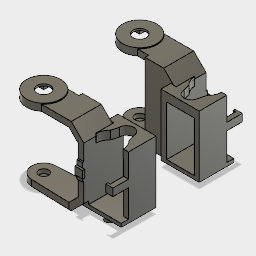
servo_bracket_knee_mirror (Autodesk Fusion 360 design; units mm, degrees)
Autodesk Fusion 360 part; units mm, degrees
sketch "スケッチ1" plane through (0, 0, 0) normal (0, 1, 0) x (1, 0, 0)
  circle A0 centre (0, 0) radius 5.55
  circle A1 centre (0, 0) radius 2.75
  line L0 (2.75, 2.75) -> (-2.75, 2.75)
  line L1 (-2.75, 2.75) -> (-2.75, -2.75)
  line L2 (-2.75, -2.75) -> (2.75, -2.75)
  line L3 (2.75, -2.75) -> (2.75, 2.75)
  line L4 (2.75, 2.75) -> (-2.75, -2.75) construction
  line L5 (-2.75, 2.75) -> (2.75, -2.75) construction
  line L6 (-2.75, 2.75) -> (-4.8208, 2.75)
  line L7 (-2.75, -2.75) -> (-4.8208, -2.75)
  line L8 (-2.75, 2.75) -> (-2.75, 4.8208)
  line L9 (-2.75, -2.75) -> (-2.75, -4.8208)
  line L10 (2.75, -2.75) -> (4.8208, -2.75)
  line L11 (2.75, -2.75) -> (2.75, -4.8208)
  line L12 (2.75, 2.75) -> (4.8208, 2.75)
  line L13 (2.75, 2.75) -> (2.75, 4.8208)
  dimension "d1" = 11.1
  dimension "d2" = 5.5
  dimension "d3" = 5.5
  dimension "d4" = 5.5
  constraint concentric A0 A1
  constraint perpendicular L0 L1
  constraint parallel L0 L2
  constraint parallel L1 L3
  constraint horizontal L0
  constraint coincident L4
  constraint coincident L5
  constraint coincident A0
  constraint perpendicular L1 L6
  constraint perpendicular L1 L7
  constraint perpendicular L7 L8
  constraint perpendicular L7 L9
  constraint perpendicular L9 L10
  constraint perpendicular L10 L11
  constraint perpendicular L11 L12
  constraint perpendicular L12 L13
  measures "d1" diameter of A0
  measures "d2" diameter of A1
sketch "スケッチ2" plane through (0, 0, 0) normal (0, 1, 0) x (1, 0, 0)
  circle A0 centre (0, 0) radius 7.15
  line L0 (5.5, 5.5) -> (-5.5, 5.5)
  line L1 (-5.5, 5.5) -> (-5.5, -5.5)
  line L2 (-5.5, -5.5) -> (5.5, -5.5)
  line L3 (5.5, -5.5) -> (5.5, 5.5)
  line L4 (5.5, 5.5) -> (-5.5, -5.5) construction
  line L5 (-5.5, 5.5) -> (5.5, -5.5) construction
  line L6 (0, 0) -> (22.2, 0)
  line L7 (5.5, -5.5) -> (5.5, 5.5)
  line L8 (5.5, 5.5) -> (22.2, 5.5)
  line L9 (22.2, 5.5) -> (22.2, -5.5)
  line L10 (22.2, -5.5) -> (5.5, -5.5)
  line L11 (22.2, -5.5) -> (19.88, -5.5)
  line L12 (19.88, -5.5) -> (19.88, 5.5)
  line L13 (19.88, 5.5) -> (22.2, 5.5)
  line L14 (22.2, 5.5) -> (22.2, -5.5)
  dimension "d5" = 14.3
  dimension "d6" = 11
  dimension "d7" = 11
  dimension "d8" = 22.2
  dimension "d9" = 2.32
  constraint perpendicular L0 L1
  constraint parallel L0 L2
  constraint parallel L1 L3
  constraint horizontal L0
  constraint coincident L4
  constraint coincident L5
  constraint perpendicular L7 L8
  constraint parallel L7 L9
  constraint parallel L8 L10
  constraint horizontal L11
  constraint vertical L12
  constraint horizontal L13
  measures "d5" diameter of A0
extrude "押し出し1" add sketch "スケッチ2" against normal blind 3 contours A0 L3 L6 L7 | A0 L3 L6 L7 | A0 L0 L1 L2 L3 L7 | A0 L0 | A0 L2 | A0 L1 makes body 1
extrude "押し出し2" cut sketch "スケッチ1" against normal blind 5.5 contours A0 L3 L10 L12 | A0 L0 L8 L13 | A1 L0 L3 | A0 L2 L9 L11 | A1 L2 L3 | A1 | A1 L0 L1 | A1 L1 L2 | A0 L1 L6 L7 bodies 1
extrude "押し出し3" add sketch "スケッチ1" against normal blind 0.8 contours A0 L3 L10 L12 | A0 L0 L8 L13 | A1 L0 L3 | A0 L2 L9 L11 | A1 L2 L3 | A1 L0 L1 | A1 L1 L2 | A0 L1 L6 L7 bodies 1
extrude "押し出し4" add sketch "スケッチ2" against normal blind 3 contours A0 L3 L6 L7 L10 L12 | A0 L3 L6 L7 L8 L12 | A0 L0 L3 L7 | A0 L2 L3 L7 bodies 1
extrude "押し出し5" add sketch "スケッチ2" against normal blind 32.7 contours L6 L8 L9 L12 L13 L14 | L6 L9 L10 L11 L12 L14 bodies 1
extrude "押し出し6" cut sketch "スケッチ2" against normal blind 0.4 contours A0 L3 L6 L7 L10 L12 | A0 L3 L6 L7 L8 L12 | A0 L0 L3 L7 | A0 L2 L3 L7 | L6 L8 L9 L12 L13 L14 | L6 L9 L10 L11 L12 L14 bodies 1
ref_plane "作業平面1" through (0, -32.7, 0) normal (0, 1, 0) x (1, 0, 0)
sketch "スケッチ3" plane through (0, -32.7, 0) normal (0, 1, 0) x (1, 0, 0)
  circle A0 centre (0, 0) radius 2
  circle A1 centre (0, 0) radius 5
  line L0 (0, 0) -> (16, 0)
  line L1 (16, 0) -> (16, 5.5)
  line L2 (16, 5.5) -> (-0.1554, 4.9976)
  line L3 (16, 5.5) -> (19.88, 5.5)
  line L4 (19.88, 5.5) -> (19.88, -5.5)
  line L5 (19.88, -5.5) -> (16, -5.5)
  line L6 (16, -5.5) -> (16, 0)
  line L7 (19.88, -5.5) -> (9.2, -5.5)
  line L8 (19.88, -5.5) -> (30.56, -5.5) construction
  line L9 (9.2, -5.5) -> (-0.2675, -4.9928)
  dimension "d23" = 4
  dimension "d24" = 10
  dimension "d25" = 16
  dimension "d26" = 180
  dimension "d27" = 10.68
  constraint perpendicular L0 L1
  constraint coincident A1
  constraint tangent A1 L2
  constraint perpendicular L1 L3
  constraint perpendicular L4 L5
  constraint horizontal L8
  constraint tangent A1 L9
  measures "d23" diameter of A0
  measures "d24" diameter of A1
  measures "d26" angle of L7 L8
extrude "押し出し7" add sketch "スケッチ3" along normal blind 2.6 bodies 1
extrude "押し出し8" add sketch "スケッチ3" along normal blind 0.8 contours A0 bodies 1
sketch "スケッチ4" plane through (0, 0, 0) normal (0, 1, 0) x (1, 0, 0)
  line L0 (22.2, -5.5) -> (22.2, -7)
  line L1 (22.2, -5.5) -> (23.7, -5.5) construction
  line L2 (22.2, -7) -> (9.2, -7)
  line L3 (22.2, -7) -> (35.2, -7) construction
  line L4 (9.2, -7) -> (9.2, -5.5)
  line L5 (9.2, -7) -> (9.2, -5.5)
  line L6 (22.2, -5.5) -> (9.2, -5.5)
  dimension "d32" = 90
  dimension "d33" = 1.5
  dimension "d34" = 180
  dimension "d35" = 13
  constraint horizontal L1
  constraint horizontal L3
  measures "d32" angle of L0 L1
  measures "d34" angle of L2 L3
extrude "押し出し9" add sketch "スケッチ4" against normal blind 32.7 bodies 1
extrude "押し出し10" cut sketch "スケッチ4" against normal blind 0.4 bodies 1
chamfer "面取り1" distance 3.88 angle 45 2 edges at (19.88, -3, 0) (19.88, -30.1, 0) on bodies 1
chamfer "面取り2" distance 5.2 angle 45 2 edges at (22.2, -0.4, 0.75) (22.2, -32.7, 0.75) on bodies 1
ref_plane "作業平面2" through (22.2, -16.55, 0.75) normal (1, 0, 0) x (0, 0, 1)
sketch "スケッチ5" plane through (22.2, -16.55, 0.75) normal (1, 0, 0) x (0, 0, -1)
  line L0 (6.25, -13.55) -> (-4.75, -13.55)
  line L1 (5.7476, -13.55) -> (-4.2428, -13.55)
  line L2 (-6.25, -10.95) -> (-6.25, -16.15)
  line L3 (-2.7394, -13.55) -> (-11.2658, -13.55)
  constraint coincident L0
  constraint perpendicular L2 L3
sketch "スケッチ6" plane through (22.2, -16.55, 0.75) normal (1, 0, 0) x (0, 0, -1)
  line L0 (-6.25, -10.95) -> (-6.25, -16.15)
  line L1 (-6.25, -13.55) -> (-6.25, -13.75)
  line L2 (-6.25, -13.55) -> (-6.05, -13.55) construction
  line L3 (-6.25, -13.75) -> (-10.25, -13.75)
  line L4 (-6.25, -13.75) -> (-2.25, -13.75) construction
  line L5 (-10.25, -13.75) -> (-6.25, -13.75)
  line L6 (-6.25, -13.75) -> (-6.25, 12.05)
  line L7 (-6.25, 12.05) -> (-10.25, 12.05)
  line L8 (-10.25, 12.05) -> (-10.25, -13.75)
  line L9 (-6.25, -13.75) -> (4.25, -13.75)
  line L10 (4.25, -13.75) -> (4.25, -12.25)
  line L11 (4.25, -12.25) -> (-6.25, -12.25)
  line L12 (-6.25, -12.25) -> (-6.25, -13.75)
  line L13 (-6.25, 12.05) -> (1.25, 12.05)
  line L14 (1.25, 12.05) -> (1.25, 8.55)
  line L15 (1.25, 8.55) -> (-6.25, 8.55)
  line L16 (-6.25, 8.55) -> (-6.25, 12.05)
  line L17 (-6.25, 8.55) -> (-10.25, 8.55)
  line L18 (-6.25, -12.25) -> (-10.25, -12.25)
  dimension "d43" = 90
  dimension "d44" = 0.2
  dimension "d45" = 180
  dimension "d46" = 4
  dimension "d47" = 25.8
  dimension "d48" = 10.5
  dimension "d49" = 1.5
  dimension "d50" = 7.5
  dimension "d51" = 3.5
  constraint midpoint L0
  constraint horizontal L2
  constraint horizontal L4
  constraint vertical L6
  constraint horizontal L7
  constraint vertical L8
  constraint horizontal L9
  constraint vertical L10
  constraint horizontal L11
  constraint vertical L12
  constraint horizontal L13
  constraint vertical L14
  constraint horizontal L15
  constraint vertical L16
  constraint coincident L8
  constraint perpendicular L8 L17
  constraint perpendicular L8 L18
  measures "d43" angle of L1 L2
  measures "d45" angle of L3 L4
extrude "押し出し11" add sketch "スケッチ6" along normal blind 2.32 separate body contours L0 L6 L8 L17 L18 makes body 2
extrude "押し出し12" add sketch "スケッチ6" along normal blind 15.92 contours L0 L1 L6 L9 L10 L11 L12 | L0 L1 L3 L5 L6 L8 L12 L18 | L6 L7 L8 L16 L17 | L6 L13 L14 L15 L16 bodies 2
extrude "押し出し13" cut sketch "スケッチ6" along normal blind 2.32 contours L0 L1 L6 L9 L10 L11 L12 | L6 L13 L14 L15 L16 bodies 2
sketch "スケッチ7" plane through (38.12, 0, 0) normal (1, 0, 0) x (0, 0, -1)
  line L0 (0.5, -4.5) -> (-11, -4.5)
  line L1 (-11, -4.5) -> (-11, -8)
  line L2 (-11, -8) -> (0.5, -8)
  line L3 (0.5, -8) -> (0.5, -4.5)
  line L4 (-11, -4.5) -> (0.5, -4.5)
  line L5 (0.5, -4.5) -> (0.5, -30.3)
  line L6 (0.5, -30.3) -> (-11, -30.3)
  line L7 (-11, -30.3) -> (-11, -4.5)
  dimension "d58" = 11.5
  dimension "d59" = 25.8
  constraint horizontal L4
  constraint vertical L5
  constraint horizontal L6
  constraint vertical L7
extrude "押し出し14" add sketch "スケッチ7" against normal blind 2 contours L2 L5 L6 L7 bodies 2
sketch "スケッチ8" plane through (0, -4.5, 0) normal (0, 1, 0) x (-1, 0, 0)
  line L0 (-24.52, 7) -> (-22.2, 7)
  line L1 (-22.2, 7) -> (-22.2, 11)
  line L2 (-22.2, 11) -> (-38.12, 11)
  line L3 (-38.12, 11) -> (-38.12, -0.5)
  line L4 (-38.12, -0.5) -> (-24.52, -0.5)
  line L5 (-24.52, -0.5) -> (-24.52, 7)
  line L6 (-24.52, -0.5) -> (-30.32, -0.5)
  line L7 (-24.52, -0.5) -> (-18.72, -0.5) construction
  circle A0 centre (-30.32, -0.5) radius 5.6
  line L8 (-30.32, -0.5) -> (-30.32, 6.5)
  line L9 (-30.32, -0.5) -> (-37.32, -0.5) construction
  circle A1 centre (-30.32, 6.5) radius 3
  line L10 (-30.32, 6.5) -> (-27.32, 6.5)
  line L11 (-30.32, 6.5) -> (-33.32, 6.5)
  line L12 (-27.32, 6.5) -> (-26.5193, 3.6127)
  line L13 (-27.32, 6.5) -> (-24.3238, 6.5) construction
  line L14 (-33.32, 6.5) -> (-34.1207, 3.6127)
  dimension "d62" = 180
  dimension "d63" = 5.8
  dimension "d64" = 11.2
  dimension "d65" = 90
  dimension "d66" = 7
  dimension "d67" = 6
  dimension "d68" = 74.5
  dimension "d69" = 105.5
  constraint horizontal L7
  constraint horizontal L9
  constraint coincident A1
  constraint perpendicular L8 L10
  constraint parallel L10 L11
  constraint coincident A0
  constraint horizontal L13
  measures "d62" angle of L6 L7
  measures "d64" diameter of A0
  measures "d65" angle of L8 L9
  measures "d67" diameter of A1
  measures "d68" angle of L12 L13
  measures "d69" angle of L13 L14
extrude "押し出し15" cut sketch "スケッチ8" against normal blind 7.5 contours L4 L6 A0 L8 A1 | L4 A0 L8 A1 | A0 A1 L12 | A0 L8 A1 | A0 L8 A1 | A0 L8 A1 L10 | A1 L10 L11 | A0 A1 L14 | A0 L8 A1 L11 bodies 2
sketch "スケッチ9" plane through (0, -30.3, 0) normal (0, -1, 0) x (1, 0, 0)
  line L0 (38.12, -3.5) -> (38.12, 11)
  line L1 (38.12, 11) -> (22.2, 11)
  line L2 (22.2, 11) -> (22.2, 7)
  line L3 (22.2, 7) -> (24.52, 7)
  line L4 (24.52, 7) -> (24.52, -3.5)
  line L5 (24.52, -3.5) -> (38.12, -3.5)
  circle A0 centre (30.32, -0.5) radius 1.9
  dimension "d72" = 3.8
  measures "d72" diameter of A0
extrude "押し出し16" add sketch "スケッチ9" along normal blind 2.4 contours A0 bodies 2
sketch "スケッチ10" plane through (36.12, 0, 0) normal (-1, 0, 0) x (0, 0, 1)
  line L0 (-0.5, -28.8) -> (11, -28.8)
  line L1 (11, -28.8) -> (11, -8)
  line L2 (11, -8) -> (-0.5, -8)
  line L3 (-0.5, -8) -> (-0.5, -28.8)
  line L4 (-0.5, -4.5) -> (-0.5, -14.3)
  line L5 (-0.5, -4.5) -> (9.3, -4.5) construction
  line L6 (-0.5, -14.3) -> (-6.975, -14.3)
  line L7 (-6.975, -14.3) -> (-6.975, -17.4)
  line L8 (-6.975, -17.4) -> (-0.5, -17.4)
  line L9 (-0.5, -17.4) -> (-0.5, -14.3)
  line L10 (-6.975, -17.4) -> (-6.1, -17.4)
  line L11 (-6.1, -17.4) -> (-6.1, -14.3)
  line L12 (-6.1, -14.3) -> (-6.975, -14.3)
  line L13 (-6.975, -14.3) -> (-6.975, -17.4)
  dimension "d75" = 90
  dimension "d76" = 9.8
  dimension "d77" = 3.1
  dimension "d78" = 6.475
  dimension "d79" = 0.875
  constraint horizontal L5
  constraint horizontal L6
  constraint vertical L7
  constraint horizontal L8
  constraint vertical L9
  constraint horizontal L10
  constraint vertical L11
  constraint horizontal L12
  measures "d75" angle of L4 L5
extrude "押し出し17" add sketch "スケッチ10" against normal blind 2 contours L3 L6 L8 L9 L11 | L6 L7 L8 L10 L11 L12 L13 bodies 2
extrude "押し出し18" add sketch "スケッチ10" along normal blind 1 contours L6 L7 L8 L10 L11 L12 L13 bodies 2
sketch "スケッチ11" plane through (19.88, 0, 0) normal (-1, 0, 0) x (0, 0, 1)
  line L0 (-5.5, -26.22) -> (5.5, -26.22)
  line L1 (5.5, -26.22) -> (5.5, -6.88)
  line L2 (5.5, -6.88) -> (-5.5, -6.88)
  line L3 (-5.5, -6.88) -> (-5.5, -26.22)
  line L4 (-6.975, -17.4) -> (-6.1, -17.4)
  line L5 (-6.1, -17.4) -> (-6.1, -14.3)
  line L6 (-6.1, -14.3) -> (-6.975, -14.3)
  line L7 (-6.975, -14.3) -> (-6.975, -17.4)
  line L8 (-0.5, -14.3) -> (-6.975, -14.3)
  line L9 (-5.5, -14.3) -> (-5.5, -12.3)
  line L10 (-5.5, -14.3) -> (-7.5, -14.3) construction
  line L11 (-5.5, -12.3) -> (-6.1, -12.3)
  line L12 (-6.1, -12.3) -> (-6.1, -19.4)
  line L13 (-6.1, -19.4) -> (-5.5, -19.4)
  line L14 (-5.5, -19.4) -> (-5.5, -12.3)
  dimension "d84" = 90
  dimension "d85" = 2
  dimension "d86" = 7.1
  dimension "d87" = 0.6
  constraint horizontal L4
  constraint vertical L5
  constraint horizontal L6
  constraint vertical L7
  constraint coincident L3
  constraint coincident L8
  constraint horizontal L10
  constraint horizontal L11
  constraint vertical L12
  constraint horizontal L13
  constraint vertical L14
  measures "d84" angle of L9 L10
extrude "押し出し19" add sketch "スケッチ11" against normal blind 2.32 contours L3 L5 L8 L12 L13 L14 | L3 L8 L9 L11 L12 L14 | L4 L5 L6 L7 L8 L12 bodies 1
extrude "押し出し20" add sketch "スケッチ11" against normal blind 3.32 contours L4 L5 L6 L7 L8 L12 bodies 1
move_body "ボディを移動1" bodies 2 to x (1, 0, 0) y (0, 1, 0) z (0, 0, 1) at (-2.32, 0, 0)
combine "結合1" operation add target body 1 tool bodies 2
sketch "スケッチ12" plane through (0, -30.3, 0) normal (0, -1, 0) x (1, 0, 0)
  circle A0 centre (28, -0.5) radius 1.9
  line L0 (35.8, -3.5) -> (35.8, 11)
  line L1 (35.8, 11) -> (19.88, 11)
  line L2 (19.88, 11) -> (19.88, 7)
  line L3 (19.88, 7) -> (22.2, 7)
  line L4 (22.2, 7) -> (22.2, -3.5)
  line L5 (22.2, -3.5) -> (35.8, -3.5)
  line L6 (22.2, 7) -> (22.2, -3.5)
  line L7 (22.2, -3.5) -> (19.477, -3.5)
  line L8 (19.477, -3.5) -> (19.477, 7)
  line L9 (19.477, 7) -> (22.2, 7)
  dimension "d94" = 2.723
  constraint perpendicular L6 L7
  constraint parallel L6 L8
  constraint parallel L7 L9
extrude "押し出し21" add sketch "スケッチ12" against normal blind 3 contours L3 L4 L6 L7 L8 L9 bodies 1
ref_plane "作業平面3" through (27.84, -17.4, 20) normal (0, 0, 1) x (0, -1, 0)
mirror "ミラー1" about plane through (27.84, -17.4, 20) normal (0, 0, 1) of bodies 1 makes body 3
